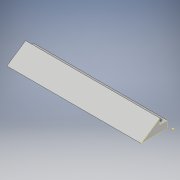
# Autodesk Inventor part: Ramp version 1
Saved by Autodesk Inventor 2019 (Build 230136000, 136)
## iProperties
Created: 2019-01-23
Part Number: Ramp version 1
Material: Generic
Document SubType Name: Modeling
Designer: mrhftc
Density: 1 g/cm^3
Appearance: Default
Author: mrhftc
Autodesk Inventor part; units mm, degrees
ref_plane "YZ Plane" through (0, 0, 0) normal (1, 0, 0) x (0, 1, 0)
sketch "Sketch1" plane through (0, 0, 0) normal (0, 1, 0) x (-1, 0, 0)
  line L0 (60.1434, 43.7027) -> (-87.3566, 43.7027)
  line L1 (-87.3566, 43.7027) -> (-87.3566, 5.6027)
  line L2 (-87.3566, 5.6027) -> (60.1434, 5.6027)
  line L3 (60.1434, 5.6027) -> (60.1434, 43.7027)
  point P0 (0, 0)
  dimension "d0" = 147.5
  dimension "d1" = 38.1
  constraints: 8 end point, 2 parallel, 1 horizontal, 1 perpendicular
  measures "d0" distance between parallel lines of L1 L3
  measures "d1" distance between parallel lines of L2 L0
extrude "Extrusion1" add sketch "Sketch1" along normal blind 19.05
ref_plane "Work Plane1" through (87.3566, 19.05, 5.6027) normal (0, -0.9396926, -0.3420201) x (-1, 0, 0)
sketch "Sketch2" plane through (87.3566, 19.05, 5.6027) normal (0, -0.9396926, -0.3420201) x (-1, 0, 0)
  line L0 (147.5, -42.3178) -> (147.5, -35.8023) construction
  line L1 (0, -35.8023) -> (0, 0) construction
  line L2 (147.5, -40.4915) -> (0, -40.4915)
  line L3 (0, -40.4915) -> (0, 0)
  line L4 (0, 0) -> (147.5, 0)
  line L5 (147.5, 0) -> (147.5, -40.4915)
  point P0 (87.3566, -1.2507)
  constraints: 8 end point, 2 parallel, 1 horizontal, 1 perpendicular, 1 point on line
extrude "Extrusion2" add sketch "Sketch2" against normal blind 19.05
sketch "Sketch3" plane through (87.3566, 36.9511, 12.1182) normal (0, 0.9396926, 0.3420201) x (1, 0, 0)
  line L0 (0, -40.4915) -> (-147.5, -40.4915) construction
  line L1 (0, -6.5155) -> (0, 0) construction
  line L2 (-147.5, -40.4915) -> (0, -40.4915)
  line L3 (0, -40.4915) -> (0, 0)
  line L4 (0, 0) -> (-147.5, 0)
  line L5 (-147.5, 0) -> (-147.5, -40.4915)
  point P0 (-87.3566, -1.2507)
  constraints: 8 end point, 2 parallel, 1 horizontal, 1 perpendicular
extrude "Extrusion3" cut sketch "Sketch3" against normal blind 19.05
ref_plane "Work Plane2" through (-79.1934, 19.05, 5.6027) normal (0, 1, 0) x (1, 0, 0)
fillet "Fillet2" radius 3.175 5 edges at (13.6066, 5.3397, 43.7027) (13.6066, 0, 43.7027) (-60.1434, 0, 24.6527) (13.6066, 0, 5.6027) (87.3566, 0, 24.6527)
fillet "Fillet3" radius 3.175 1 edges at (13.6066, 19.0479, 5.6027)
sketch "Sketch12" plane through (87.3566, 3.175, 43.7027) normal (1, 0, 0) x (0, 0, -1)
  line L0 (38.121, 6.8749) -> (30.121, 6.8749)
  line L1 (30.121, 6.8749) -> (30.121, 14.8749)
  line L2 (30.121, 14.8749) -> (38.121, 14.8749)
  line L3 (38.121, 14.8749) -> (38.121, 6.8749)
  dimension "d36" = 8
  dimension "d37" = 8
  constraints: 8 end point
  measures "d36" distance between parallel lines of L1 L3
  measures "d37" distance between parallel lines of L0 L2
extrude "Extrusion9" cut sketch "Sketch12" against normal through all
sketch "Sketch13" plane through (87.3566, 10.0499, 13.5817) normal (0, 1, 0) x (1, 0, 0)
  line L0 (-73.75, 7.979) -> (-73.75, -0.1527)
  circle A0 centre (-73.75, 3.9895) radius 2.1
  circle A1 centre (-81.75, 3.9895) radius 2.1
  circle A2 centre (-89.75, 3.9895) radius 2.1
  circle A3 centre (-97.75, 3.9895) radius 2.1
  circle A4 centre (-105.75, 3.9895) radius 2.1
  circle A5 centre (-113.75, 3.9895) radius 2.1
  circle A6 centre (-121.75, 3.9895) radius 2.1
  circle A7 centre (-129.75, 3.9895) radius 2.1
  circle A8 centre (-137.75, 3.9895) radius 2.1
  circle A9 centre (-65.75, 3.9895) radius 2.1
  circle A10 centre (-57.75, 3.9895) radius 2.1
  circle A11 centre (-49.75, 3.9895) radius 2.1
  circle A12 centre (-41.75, 3.9895) radius 2.1
  circle A13 centre (-33.75, 3.9895) radius 2.1
  circle A14 centre (-25.75, 3.9895) radius 2.1
  circle A15 centre (-17.75, 3.9895) radius 2.1
  circle A16 centre (-9.75, 3.9895) radius 2.1
  constraints: 17 centre point, 8 symmetric about line, 2 end point, 1 vertical, 8 other
extrude "Extrusion10" cut sketch "Sketch13" against normal through all
sketch "Sketch14" plane through (87.3566, 3.175, 43.7027) normal (1, 0, 0) x (0, 0, -1)
  line L0 (-30.4844, 21.6462) -> (52.8728, 21.6462)
  line L1 (52.8728, 21.6462) -> (52.8728, -12.2101)
  line L2 (52.8728, -12.2101) -> (-30.4844, -12.2101)
  line L3 (-30.4844, -12.2101) -> (-30.4844, 21.6462)
  point P0 (43.7027, -3.175)
  constraints: 8 end point, 2 parallel, 1 horizontal, 1 perpendicular
extrude "Extrusion11" cut sketch "Sketch14" against normal blind 5.08
sketch "Sketch15" plane through (-60.1434, 3.175, 43.7027) normal (-1, 0, 0) x (0, 0, 1)
  line L0 (33.6252, 94.5491) -> (-79.5372, 94.5491)
  line L1 (-79.5372, 94.5491) -> (-79.5372, -54.7848)
  line L2 (-79.5372, -54.7848) -> (33.6252, -54.7848)
  line L3 (33.6252, -54.7848) -> (33.6252, 94.5491)
  point P0 (-43.7027, -3.175)
  constraints: 8 end point, 2 parallel, 1 horizontal, 1 perpendicular
extrude "Extrusion12" cut sketch "Sketch15" against normal blind 5.08
sketch "Sketch16" plane through (82.2766, 3.175, 43.7027) normal (1, 0, 0) x (0, 0, -1)
  arc A0 (34.925, -3.175) -> (38.1, 0) centre (34.925, 0) ccw construction
  line L0 (-8.1127, -3.175) -> (38.1, -3.175)
  line L1 (38.1, -3.175) -> (38.1, 0)
  line L2 (38.1, 0) -> (-8.1127, 0)
  line L3 (-8.1127, 0) -> (-8.1127, -3.175)
  line L4 (0, 1.4623) -> (0, 0) construction
  line L5 (30.121, 12.9709) -> (11.0545, 0)
  line L6 (11.2811, 0) -> (-2.3132, 0)
  line L7 (-2.3132, 0) -> (0.9299, 12.0527)
  line L8 (0.0505, 2.0261) -> (30.121, 12.9709) construction
  line L9 (0.9299, 12.0527) -> (30.121, 12.9709)
  point P0 (43.7027, -3.175)
  point P1 (0, 0.7312)
  constraints: 16 end point, 3 point on line, 2 parallel, 1 horizontal, 1 midpoint, 1 perpendicular, 1 point on circle
extrude "Extrusion14" cut sketch "Sketch16" against normal through all
sketch "Sketch17" plane through (82.2766, 3.175, 43.7027) normal (1, 0, 0) x (0, 0, -1)
  line L0 (30.121, 12.9709) -> (11.0545, 0) construction
  line L1 (11.0545, 0) -> (38.1, 0) construction
  line L2 (38.1, 6.8749) -> (38.1, 0) construction
  line L3 (30.121, 6.8749) -> (38.1, 6.8749) construction
  line L4 (30.121, 12.9709) -> (30.121, 6.8749) construction
  point P0 (43.7027, -3.175)
body "Solid1"
